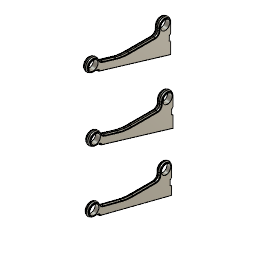
Shelf Brackets Filament Spool Holders A6 (Autodesk Fusion 360 design; units mm, degrees)
Autodesk Fusion 360 part; units mm, degrees
(part 1 of 2)
sketch "Sketch1" plane through (0, 0, 0) normal (1, 0, 0) x (0, 1, 0) in component "GROUND Spool Bambu Lab 1kg"
  circle A0 centre (0, 0) radius 27.5
  circle A1 centre (0, 0) radius 25
  circle A2 centre (0, 0) radius 100
  circle A3 centre (0, 0) radius 44.5
  circle A4 centre (0, 0) radius 41
  dimension "d1" = 55
  dimension "d2" = 50
  dimension "d3" = 200
  dimension "d4" = 89
  dimension "d5" = 82
  constraint coincident A0.centre A1.centre
  constraint concentric A1 A2
  constraint concentric A0 A3
  constraint concentric A0 A4
  measures "d1" diameter of A0
  measures "d2" diameter of A1
  measures "d3" diameter of A2
  measures "d4" diameter of A3
  measures "d5" diameter of A4
extrude "Extrude1" add sketch "Sketch1" against normal blind 3.5 contours A0 | A2 | A3 | A4 picked at (26.471206, -2.60824) picked at (80.962018, -7.178869) picked at (43.015012, -4.247705) picked at (36.347355, -2.036911) makes body 1 in component "GROUND Spool Bambu Lab 1kg"
extrude "Extrude2" add sketch "Sketch1" along normal blind 3.5 from surface at 60 separate body contours A0 | A2 | A3 | A4 picked at (26.471206, -2.60824) picked at (80.962018, -7.178869) picked at (43.015012, -4.247705) picked at (36.347355, -2.036911) makes body 2 in component "GROUND Spool Bambu Lab 1kg"
extrude "Extrude3" add sketch "Sketch1" along normal blind 63.5 contours A4 picked at (36.347355, -2.036911) bodies 1 2 in component "GROUND Spool Bambu Lab 1kg"
extrude "Extrude4" add sketch "Sketch1" along normal blind 32 contours A0 picked at (26.471206, -2.60824) bodies 1 in component "GROUND Spool Bambu Lab 1kg"
extrude "Extrude5" add sketch "Sketch1" along normal blind 60 separate body contours A3 picked at (43.015012, -4.247705) makes body 3 in component "GROUND Spool Bambu Lab 1kg"
sketch "Sketch1 (2)" plane through (0, 0, 0) normal (1, 0, 0) x (0, 1, 0) in component "Spool Bambu Lab 1kg (1)"
  circle A0 centre (0, 0) radius 27.5
  circle A1 centre (0, 0) radius 25
  circle A2 centre (0, 0) radius 100
  circle A3 centre (0, 0) radius 44.5
  circle A4 centre (0, 0) radius 41
  dimension "d1_1" = 55
  dimension "d2_1" = 50
  dimension "d3_1" = 200
  dimension "d4_1" = 89
  dimension "d5_1" = 82
  constraint coincident A0.centre A1.centre
  constraint concentric A1 A2
  constraint concentric A0 A3
  constraint concentric A0 A4
  measures "d1_1" diameter of A0
  measures "d2_1" diameter of A1
  measures "d3_1" diameter of A2
  measures "d4_1" diameter of A3
  measures "d5_1" diameter of A4
extrude "Extrude1'" add sketch "Sketch1 (2)" against normal blind 3.5 separate body contours A0 | A2 | A3 | A4 picked at (26.471206, -2.60824) picked at (80.962018, -7.178869) picked at (43.015012, -4.247705) picked at (36.347355, -2.036911) makes body 4 in component "Spool Bambu Lab 1kg (1)"
extrude "Extrude2'" add sketch "Sketch1 (2)" along normal blind 3.5 from surface at 60 separate body contours A0 | A2 | A3 | A4 picked at (26.471206, -2.60824) picked at (80.962018, -7.178869) picked at (43.015012, -4.247705) picked at (36.347355, -2.036911) makes body 5 in component "Spool Bambu Lab 1kg (1)"
extrude "Extrude3'" add sketch "Sketch1 (2)" along normal blind 63.5 contours A4 picked at (36.347355, -2.036911) bodies 4 5 in component "Spool Bambu Lab 1kg (1)"
extrude "Extrude4'" add sketch "Sketch1 (2)" along normal blind 32 contours A0 picked at (26.471206, -2.60824) bodies 4 in component "Spool Bambu Lab 1kg (1)"
extrude "Extrude5'" add sketch "Sketch1 (2)" along normal blind 60 separate body contours A3 picked at (43.015012, -4.247705) makes body 6 in component "Spool Bambu Lab 1kg (1)"
sketch "Sketch1 (3)" plane through (0, 0, 0) normal (1, 0, 0) x (0, 1, 0) in component "Box Bambu Lab Refill"
  line L0 (100, -97.5) -> (-100, -97.5)
  line L1 (-100, -97.5) -> (-100, 97.5)
  line L2 (-100, 97.5) -> (100, 97.5)
  line L3 (100, 97.5) -> (100, -97.5)
  line L4 (100, -97.5) -> (-100, 97.5) construction
  line L5 (-100, -97.5) -> (100, 97.5) construction
  dimension "d17" = 200
  dimension "d18" = 195
  constraint horizontal L0
  constraint perpendicular L0 L1
  constraint parallel L0 L2
  constraint parallel L1 L3
  constraint coincident L4 origin
  constraint coincident L5 origin
  measures "d17" distance of L1.end L2.end
  measures "d18" distance of L0.end L1.end
extrude "Extrude1''" add sketch "Sketch1 (3)" along normal blind 66 separate body contours L0 L1 L2 L3 picked at (33.333333, -32.5) makes body 7 in component "Box Bambu Lab Refill"
sketch "Sketch1 (4)" plane through (0, 0, 0) normal (1, 0, 0) x (0, 1, 0) in component "Box Bambu Lab with Spool"
  line L0 (110, -103) -> (-110, -103)
  line L1 (-110, -103) -> (-110, 103)
  line L2 (-110, 103) -> (110, 103)
  line L3 (110, 103) -> (110, -103)
  line L4 (110, -103) -> (-110, 103) construction
  line L5 (-110, -103) -> (110, 103) construction
  dimension "d17_1" = 220
  dimension "d18_1" = 206
  constraint horizontal L0
  constraint perpendicular L0 L1
  constraint parallel L0 L2
  constraint parallel L1 L3
  constraint coincident L4 origin
  constraint coincident L5 origin
  measures "d17_1" distance of L1.end L2.end
  measures "d18_1" distance of L0.end L1.end
extrude "Extrude1'''" add sketch "Sketch1 (4)" along normal blind 70 separate body contours L0 L1 L2 L3 picked at (36.666667, 34.333333) makes body 8 in component "Box Bambu Lab with Spool"
sketch "Sketch1 (5)" plane through (0, 0, 0) normal (1, 0, 0) x (0, 1, 0) in component "Box Polymaker"
  line L0 (111.5, -103.5) -> (-111.5, -103.5)
  line L1 (-111.5, -103.5) -> (-111.5, 103.5)
  line L2 (-111.5, 103.5) -> (111.5, 103.5)
  line L3 (111.5, 103.5) -> (111.5, -103.5)
  line L4 (111.5, -103.5) -> (-111.5, 103.5) construction
  line L5 (-111.5, -103.5) -> (111.5, 103.5) construction
  dimension "d25" = 223
  dimension "d26" = 207
  constraint horizontal L0
  constraint perpendicular L0 L1
  constraint parallel L0 L2
  constraint parallel L1 L3
  constraint coincident L4 origin
  constraint coincident L5 origin
  measures "d25" distance of L1.end L2.end
  measures "d26" distance of L0.end L1.end
extrude "Extrude1''''" add sketch "Sketch1 (5)" along normal blind 74 separate body contours L0 L1 L2 L3 picked at (37.166667, -34.5) makes body 9 in component "Box Polymaker"
sketch "Sketch1 (6)" plane through (0, 0, 0) normal (0, 1, 0) x (1, 0, 0) in component "Shelf Vertical Track 48\""
  line L0 (11.5, -624) -> (-11.5, -624)
  line L1 (-11.5, -624) -> (-11.5, 624)
  line L2 (-11.5, 624) -> (11.5, 624)
  line L3 (11.5, 624) -> (11.5, -624)
  line L4 (11.5, -624) -> (-11.5, 624) construction
  line L5 (-11.5, -624) -> (11.5, 624) construction
  line L6 (9.6, -624) -> (9.6, 624)
  line L7 (-9.6, 624) -> (-9.6, -624)
  line L8 (-3.75, -616.3) -> (-3.75, -600.3)
  arc A0 (-3.75, -600.3) -> (-6.75, -600.3) centre (-5.25, -600.3) ccw
  line L9 (-6.75, -600.3) -> (-6.75, -616.3)
  arc A1 (-6.75, -616.3) -> (-3.75, -616.3) centre (-5.25, -616.3) ccw
  line L10 (-5.25, -616.3) -> (-5.25, -600.3) construction
  line L11 (3.75, -600.3) -> (3.75, -616.3)
  line L12 (5.25, -616.3) -> (5.25, -600.3) construction
  arc A2 (3.75, -616.3) -> (6.75, -616.3) centre (5.25, -616.3) ccw
  line L13 (6.75, -616.3) -> (6.75, -600.3)
  arc A3 (6.75, -600.3) -> (3.75, -600.3) centre (5.25, -600.3) ccw
  line L14 (-5.25, -616.3) -> (5.25, -616.3) construction
  line L15 (0, -624) -> (0, 624) construction
  circle A4 centre (0, -591) radius 3
  circle A5 centre (0, -336.5) radius 3
  circle A6 centre (0, 107.5) radius 3
  circle A7 centre (0, 552) radius 3
  point P0 (0, -616.3)
  point P1 (0, -624)
  dimension "d29" = 23
  dimension "d30" = 1248
  dimension "d31" = 1.9
  dimension "d32" = 1.9
  dimension "d34" = 3
  dimension "d35" = 16
  dimension "d36" = 7.7
  dimension "d37" = 3
  dimension "d38" = 16
  dimension "d39" = 10.5
  dimension "d40" = 6
  dimension "d41" = 33
  dimension "d42" = 6
  dimension "d43" = 287.5
  dimension "d45" = 6
  dimension "d46" = 731.5
  dimension "d47" = 6
  dimension "d48" = 72
  constraint horizontal L0
  constraint perpendicular L0 L1
  constraint parallel L0 L2
  constraint parallel L1 L3
  constraint coincident L4 origin
  constraint coincident L5 origin
  constraint coincident L0 L6.start
  constraint coincident L2 L6.end
  constraint perpendicular L2 L6
  constraint coincident L2 L7.start
  constraint coincident L0 L7.end
  constraint perpendicular L0 L7
  constraint tangent L8 A0
  constraint tangent A0 L9
  constraint parallel L8 L9
  constraint tangent L9 A1
  constraint tangent L8 A1
  constraint vertical L10
  constraint tangent L13 A3
  constraint tangent L11 A3
  constraint parallel L11 L13
  constraint tangent L11 A2
  constraint tangent A2 L13
  constraint vertical L12
  constraint coincident A1.centre L10.start
  constraint coincident L12.start A2.centre
  constraint horizontal L14
  constraint midpoint L14 P0
  constraint midpoint L0 P1
  constraint coincident P1 L15.start
  constraint midpoint L2 L15.end
  constraint coincident P0 L15
  constraint coincident L15 A4.centre
  constraint coincident L15 A5.centre
  constraint coincident L15 A6.centre
  constraint coincident L15 A7.centre
  measures "d29" distance of L1.end L2.end
  measures "d30" distance of L0.end L1.end
  measures "d31" distance of L1 L7
  measures "d32" distance of L3 L6
  measures "d34" distance of L8 L9
  measures "d35" distance of A1.centre A0.centre
  measures "d36" distance of L0 A1.centre
  measures "d37" distance of L11 L13
  measures "d38" distance of L12.start L12.end
  measures "d39" distance of A1.centre L12.start
  measures "d40" diameter of A4
  measures "d41" distance of L0 A4.centre
  measures "d42" diameter of A5
  measures "d43" distance of L0 A5.centre
  measures "d45" diameter of A6
  measures "d46" distance of L0 A6.centre
  measures "d47" diameter of A7
  measures "d48" distance of L2 A7.centre
extrude "Extrude1'''''" add sketch "Sketch1 (6)" against normal blind 1.9 separate body contours L0 L2 L3 L6 | L0 L2 L6 L7 | L0 L1 L2 L7 picked at (10.866667, 208) picked at (0, 601) picked at (-10.233333, 208) makes body 10 in component "Shelf Vertical Track 48\""
extrude "Extrude2''" add sketch "Sketch1 (6)" along normal blind 15 contours L0 L2 L3 L6 | L0 L1 L2 L7 picked at (10.866667, 208) picked at (-10.233333, 208) bodies 10 in component "Shelf Vertical Track 48\""
fillet "Fillet1" radius 2 2 edges at (-11.5, -1.9, 0) (11.5, -1.9, 0) on bodies 10 in component "Shelf Vertical Track 48\""
fillet "Fillet2" radius 0.6 2 edges at (-9.6, 0, 0) (9.6, 0, 0) on bodies 10 in component "Shelf Vertical Track 48\""
pattern_linear "R-Pattern1" count 39 spacing 31.757896 along (0, 0, -1) of 8 faces at (6.75, -1.266667, 610.966667) (4.436181, -1.266667, 617.560039) (6.063819, -1.266667, 599.039961) (-4.436181, -1.266667, 599.039961) (-3.75, -1.266667, 610.966667) (-6.063819, -1.266667, 617.560039) (-6.75, -1.266667, 605.633333) (3.75, -1.266667, 605.633333) on bodies 10 in component "Shelf Vertical Track 48\""
sketch "Sketch1 (7)" plane through (0, 0, 0) normal (1, 0, 0) x (0, 1, 0) in component "Shelf Bracket 9.53\""
  line L0 (0, 0) -> (-265, 0)
  line L1 (0, 0) -> (0, -56) construction
  line L2 (0, -56) -> (-265, 0)
  line L3 (-242, 0) -> (-242, -4.860377)
  line L4 (-10, 0) -> (-10, -53.886792) construction
  line L5 (-12, 0) -> (-12, -53.464151) construction
  line L6 (-13, 0) -> (-13, -53.25283) construction
  line L7 (-11, 0) -> (-11, -53.675472) construction
  line L8 (0, -16.675472) -> (-10, -16.675472)
  line L9 (-4.5, -42.175472) -> (-11, -42.175472)
  line L10 (-8, -25.675472) -> (-12, -25.675472)
  line L11 (-8, -25.675472) -> (-4.5, -42.175472)
  line L12 (-12, -25.675472) -> (-12, -18.675472)
  line L13 (-13, -16.675472) -> (-13, -11.675472)
  line L14 (-13, -11.675472) -> (-10, -11.675472)
  line L15 (-10, -11.675472) -> (-10, -16.675472)
  line L16 (-12, -18.675472) -> (-13, -16.675472)
  line L17 (-11, -42.175472) -> (-11, -53.675472)
  line L18 (-255.810366, 0) -> (-11, -51.733511)
  line L19 (0, 0) -> (0, -16.675472)
  line L20 (-243.9, 0) -> (-243.9, -4.458868)
  point P0 (-242, 0)
  dimension "d65" = 265
  dimension "d66" = 56
  dimension "d67" = 242
  dimension "d68" = 10
  dimension "d69" = 12
  dimension "d70" = 13
  dimension "d71" = 11
  dimension "d72" = 37
  dimension "d73" = 11.5
  dimension "d74" = 28
  dimension "d75" = 6.5
  dimension "d76" = 4
  dimension "d77" = 7
  dimension "d78" = 9
  dimension "d79" = 14
  dimension "d82" = 1.9
  dimension "d88" = 1.9
  constraint coincident L0.start L1.start
  constraint horizontal L0
  constraint perpendicular L0 L1
  constraint coincident L0 P0
  constraint coincident P0 L3.start
  constraint perpendicular L0 L3
  constraint coincident L0 L4.start
  constraint perpendicular L0 L4
  constraint coincident L0 L5.start
  constraint perpendicular L0 L5
  constraint coincident L0 L6.start
  constraint perpendicular L0 L6
  constraint coincident L0 L7.start
  constraint perpendicular L0 L7
  constraint perpendicular L4 L8
  constraint perpendicular L7 L9
  constraint perpendicular L5 L10
  constraint perpendicular L10 L12
  constraint perpendicular L4 L14
  constraint parallel L2 L18
  constraint coincident L0 L20.start
  constraint perpendicular L0 L20
  measures "d65" distance of L0.start L0.end
  measures "d66" distance of L0.start L1.end
  measures "d67" distance of L1 P0
  measures "d68" distance of L1 L4
  measures "d69" distance of L1 L5
  measures "d70" distance of L1 L6
  measures "d71" distance of L1 L7
  measures "d82" distance of L2 L18
  measures "d88" distance of L3 L20
extrude "Extrude1''''''" add sketch "Sketch1 (7)" against normal blind 1.9 separate body contours L0 L3 L8 L9 L10 L11 L12 L13 L14 L15 L16 L17 L18 L19 | L0 L3 L18 L20 | L2 L3 L17 L18 | L2 L3 L18 L20 picked at (-88.333333, -23.589787) picked at (-242.633333, -1.811775) picked at (-165, -19.837435) picked at (-242.633333, -4.079221) makes body 11 in component "Shelf Bracket 9.53\""
extrude "Extrude2'''" add sketch "Sketch1 (7)" along normal blind 9.94 contours L0 L3 L18 L20 | L2 L3 L17 L18 | L2 L3 L18 L20 picked at (-242.633333, -1.811775) picked at (-165, -19.837435) picked at (-242.633333, -4.079221) bodies 11 in component "Shelf Bracket 9.53\""
extrude "Extrude3''" add sketch "Sketch1 (7)" along normal blind 1.9 from surface at 9.94 contours L0 L3 L8 L9 L10 L11 L12 L13 L14 L15 L16 L17 L18 L19 | L0 L3 L18 L20 | L2 L3 L17 L18 | L2 L3 L18 L20 picked at (-88.333333, -23.589787) picked at (-242.633333, -1.811775) picked at (-165, -19.837435) picked at (-242.633333, -4.079221) bodies 11 in component "Shelf Bracket 9.53\""
fillet "Fillet1'" radius 4 1 edges at (4.97, -242, -2.918417) on bodies 11 in component "Shelf Bracket 9.53\""
fillet "Fillet2'" radius 6 1 edges at (4.97, -243.9, -4.458868) on bodies 11 in component "Shelf Bracket 9.53\""
fillet "Fillet3" radius 1.8 4 edges at (10.89, 0, -16.675472) (-0.95, 0, -16.675472) (10.89, -10, -16.675472) (-0.95, -10, -16.675472) on bodies 11 in component "Shelf Bracket 9.53\""
fillet "Fillet4" radius 7 2 edges at (-0.95, 0, 0) (10.89, 0, 0) on bodies 11 in component "Shelf Bracket 9.53\""
fillet "Fillet5" radius 1.5 2 edges at (10.89, -8, -25.675472) (-0.95, -8, -25.675472) on bodies 11 in component "Shelf Bracket 9.53\""
fillet "Fillet6" radius 1.5 2 edges at (10.89, -4.5, -42.175472) (-0.95, -4.5, -42.175472) on bodies 11 in component "Shelf Bracket 9.53\""
fillet "Fillet7" radius 0.6 12 edges at (10.89, -10, -11.675472) (10.89, -13, -11.675472) (-0.95, -13, -11.675472) (-0.95, -10, -11.675472) (-0.95, -13, -16.675472) (10.89, -13, -16.675472) (10.89, -12, -18.675472) (-0.95, -12, -18.675472) (10.89, -12, -25.675472) (-0.95, -12, -25.675472) (10.89, -11, -42.175472) (-0.95, -11, -42.175472) on bodies 11 in component "Shelf Bracket 9.53\""
fillet "Fillet8" radius 0.8 1 edges at (4.97, -11, -53.675472) on bodies 11 in component "Shelf Bracket 9.53\""
sketch "Sketch2" plane through (0, -11.32809, -53.60614) normal (0, -0.206755, -0.978393) x (1, 0, 0) in component "Shelf Bracket 9.53\""
  line L0 (-1.9, 0.651389) -> (11.84, 0.651389)
  line L1 (11.84, 0.651389) -> (11.84, 232.857773)
  line L2 (11.84, 232.857773) -> (-1.9, 232.857773)
  line L3 (-1.9, 232.857773) -> (-1.9, 0.651389)
  line L4 (4.97, 232.857773) -> (4.97, 0.651389) construction
  circle A0 centre (4.97, 62.651389) radius 2
  line L5 (2.97, 163.651389) -> (2.97, 148.651389)
  arc A1 (2.97, 148.651389) -> (6.97, 148.651389) centre (4.97, 148.651389) ccw
  line L6 (6.97, 148.651389) -> (6.97, 163.651389)
  arc A2 (6.97, 163.651389) -> (2.97, 163.651389) centre (4.97, 163.651389) ccw
  line L7 (4.97, 163.651389) -> (4.97, 148.651389) construction
  dimension "d105" = 4
  dimension "d106" = 62
  dimension "d107" = 4
  dimension "d108" = 15
  dimension "d109" = 148
  constraint tangent L5 A1
  constraint tangent A1 L6
  constraint parallel L5 L6
  constraint tangent L6 A2
  constraint tangent L5 A2
  constraint parallel L4 L7
  measures "d105" diameter of A0
  measures "d107" distance of L5 L6
extrude "Extrude4''" cut sketch "Sketch2" against normal up to surface (1.9 mm away) contours A0 | L5 A1 L6 A2 picked at (5.466147, 63.005476) picked at (4.303333, 158.651389) bodies 11 in component "Shelf Bracket 9.53\""
sketch "Sketch1 (8)" plane through (0, 0, 0) normal (1, 0, 0) x (0, 1, 0) in component "Lowes Shelf Bracket 9.53\" (1)"
  line L0 (0, 0) -> (-188.527967, 0)
  line L1 (-11, -53.2) -> (-188.527967, 0)
  line L2 (-174, 0) -> (-174, -4.353612)
  line L3 (-10, 0) -> (-10, -12) construction
  line L4 (-12, 0) -> (-12, -52.900329) construction
  line L5 (-13, 0) -> (-13, -52.600658) construction
  line L6 (-11, 0) -> (-11, -53.2) construction
  line L7 (0, -16.6) -> (-10, -16.6)
  line L8 (-4.5, -42.1) -> (-11, -42.1)
  line L9 (-8, -26) -> (-12, -26)
  line L10 (-8, -26) -> (-4.5, -42.1)
  line L11 (-12, -26) -> (-12, -19)
  line L12 (-13, -17) -> (-13, -12)
  line L13 (-13, -12) -> (-10, -12)
  line L14 (-10, -12) -> (-10, -16.6)
  line L15 (-12, -19) -> (-13, -17)
  line L16 (-11, -42.1) -> (-11, -53.2)
  line L17 (-184.417312, 0) -> (-11, -51.968155)
  line L18 (0, 0) -> (0, -16.6)
  line L19 (-175.18, 0) -> (-175.18, -4)
  point P0 (-174, 0)
  point P1 (-175.18, -4)
  dimension "d75_1" = 6.5
  dimension "d76_1" = 4
  dimension "d77_1" = 7
  dimension "d78_1" = 9
  dimension "d79_1" = 14
  dimension "d82_1" = 1.18
  dimension "d88_1" = 1.18
  dimension "d198" = 4
  dimension "d199" = 53.2
  dimension "d200" = 16.6
  dimension "d201" = 12
  dimension "d202" = 42.1
  dimension "d203" = 10
  dimension "d204" = 11
  dimension "d205" = 12
  dimension "d206" = 13
  dimension "d207" = 174
  constraint coincident L0.start L18.start
  constraint horizontal L0
  constraint coincident L0 P0
  constraint coincident P0 L2.start
  constraint perpendicular L0 L2
  constraint coincident L0 L3.start
  constraint perpendicular L0 L3
  constraint coincident L0 L4.start
  constraint perpendicular L0 L4
  constraint coincident L0 L5.start
  constraint perpendicular L0 L5
  constraint coincident L0 L6.start
  constraint perpendicular L0 L6
  constraint coincident L1 L6.end
  constraint coincident L3 L7.end
  constraint perpendicular L3 L7
  constraint coincident L6 L8.end
  constraint perpendicular L6 L8
  constraint coincident L4 L9.end
  constraint perpendicular L4 L9
  constraint perpendicular L9 L11
  constraint coincident L5 L12.start
  constraint coincident L5 L12.end
  constraint coincident L3 L13.end
  constraint perpendicular L3 L13
  constraint parallel L1 L17
  constraint coincident L0 L19.start
  constraint perpendicular L0 L19
  constraint coincident L1 P1
  constraint coincident L19 P1
  constraint coincident L1.start L6
  constraint coincident L3.end L13.end
  measures "d75_1" distance of L8.start L8.end
  measures "d76_1" distance of L9.start L9.end
  measures "d77_1" distance of L9.end L11.end
  measures "d78_1" vertical distance of L9.end L12.start
  measures "d79_1" vertical distance of L9.end L12.end
  measures "d82_1" distance of L1 L17
  measures "d88_1" distance of L2 L19
  measures "d198" distance of L19.start P1
  measures "d199" distance of L0 L1.start
  measures "d200" distance of L0 L7
  measures "d201" distance of L0 L13
  measures "d202" distance of L0 L8
  measures "d203" distance of L3 L18
  measures "d204" distance of L6 L18
  measures "d205" distance of L4 L18
  measures "d206" distance of L5 L18
  measures "d207" distance of L2 L18
extrude "Extrude1'''''''" add sketch "Sketch1 (8)" against normal blind 1.18 separate body contours L0 L2 L7 L8 L9 L10 L11 L12 L13 L14 L15 L16 L17 L18 | L0 L2 L17 L19 | L1 L2 L16 L17 | L1 L2 L17 L19 picked at (-65.666667, -23.740589) picked at (-174.393333, -1.963307) picked at (-65.333333, -36.507256) picked at (-174.393333, -3.825126) makes body 12 in component "Lowes Shelf Bracket 9.53\" (1)"
extrude "Extrude2''''" add sketch "Sketch1 (8)" along normal blind 10.64 contours L0 L2 L17 L19 | L1 L2 L16 L17 | L1 L2 L17 L19 picked at (-174.393333, -1.963307) picked at (-65.333333, -36.507256) picked at (-174.393333, -3.825126) bodies 12 in component "Lowes Shelf Bracket 9.53\" (1)"
extrude "Extrude3'''" add sketch "Sketch1 (8)" along normal blind 1.18 from surface at 10.64 contours L0 L2 L7 L8 L9 L10 L11 L12 L13 L14 L15 L16 L17 L18 | L0 L2 L17 L19 | L1 L2 L16 L17 | L1 L2 L17 L19 picked at (-65.666667, -23.740589) picked at (-174.393333, -1.963307) picked at (-65.333333, -36.507256) picked at (-174.393333, -3.825126) bodies 12 in component "Lowes Shelf Bracket 9.53\" (1)"
fillet "Fillet1''" radius 4 1 edges at (5.32, -174, -3.121767) on bodies 12 in component "Lowes Shelf Bracket 9.53\" (1)"
fillet "Fillet2''" radius 6 1 edges at (5.32, -175.18, -4) on bodies 12 in component "Lowes Shelf Bracket 9.53\" (1)"
fillet "Fillet3'" radius 1.8 4 edges at (11.23, 0, -16.6) (-0.59, 0, -16.6) (11.23, -10, -16.6) (-0.59, -10, -16.6) on bodies 12 in component "Lowes Shelf Bracket 9.53\" (1)"
fillet "Fillet4'" radius 7 2 edges at (-0.59, 0, 0) (11.23, 0, 0) on bodies 12 in component "Lowes Shelf Bracket 9.53\" (1)"
fillet "Fillet5'" radius 1.5 2 edges at (11.23, -8, -26) (-0.59, -8, -26) on bodies 12 in component "Lowes Shelf Bracket 9.53\" (1)"
fillet "Fillet6'" radius 1.5 2 edges at (11.23, -4.5, -42.1) (-0.59, -4.5, -42.1) on bodies 12 in component "Lowes Shelf Bracket 9.53\" (1)"
fillet "Fillet7'" radius 0.6 12 edges at (11.23, -10, -12) (11.23, -13, -12) (-0.59, -13, -12) (-0.59, -10, -12) (-0.59, -13, -17) (11.23, -13, -17) (11.23, -12, -19) (-0.59, -12, -19) (11.23, -12, -26) (-0.59, -12, -26) (11.23, -11, -42.1) (-0.59, -11, -42.1) on bodies 12 in component "Lowes Shelf Bracket 9.53\" (1)"
fillet "Fillet8'" radius 0.8 1 edges at (5.32, -11, -53.2) on bodies 12 in component "Lowes Shelf Bracket 9.53\" (1)"
sketch "Sketch2 (2)" plane through (0, -15.535226, -51.840924) normal (0, -0.287059, -0.957913) x (1, 0, 0) in component "Lowes Shelf Bracket 9.53\" (1)"
  line L0 (-1.18, -3.659601) -> (11.82, -3.659601)
  line L1 (11.82, -3.659601) -> (11.82, 162.212706)
  line L2 (11.82, 162.212706) -> (-1.18, 162.212706)
  line L3 (-1.18, 162.212706) -> (-1.18, -3.659601)
  line L4 (5.32, 162.212706) -> (5.32, -3.659601) construction
  circle A0 centre (5.32, 41.840399) radius 2
  line L5 (3.32, 116.840399) -> (3.32, 101.840399)
  arc A1 (3.32, 101.840399) -> (7.32, 101.840399) centre (5.32, 101.840399) ccw
  line L6 (7.32, 101.840399) -> (7.32, 116.840399)
  arc A2 (7.32, 116.840399) -> (3.32, 116.840399) centre (5.32, 116.840399) ccw
  line L7 (5.32, 116.840399) -> (5.32, 101.840399) construction
  dimension "d105_1" = 4
  dimension "d106_1" = 45.5
  dimension "d107_1" = 4
  dimension "d108_1" = 15
  dimension "d109_1" = 105.5
  constraint tangent L5 A1
  constraint tangent A1 L6
  constraint parallel L5 L6
  constraint tangent L6 A2
  constraint tangent L5 A2
  constraint parallel L4 L7
  measures "d105_1" diameter of A0
  measures "d107_1" distance of L5 L6
extrude "Extrude4'''" cut sketch "Sketch2 (2)" against normal up to surface (1.18 mm away) contours A0 | L5 A1 L6 A2 picked at (5.847074, 41.218829) picked at (5.986667, 106.840399) bodies 12 in component "Lowes Shelf Bracket 9.53\" (1)"
sketch "Sketch1 (9)" plane through (0, 0, 0) normal (1, 0, 0) x (0, 1, 0) in component "Pipe Holder"
  arc A0 (-12, -18.817112) -> (-12.063344, -18.548784) centre (-12.6, -18.817112) ccw
  line L0 (-12.063344, -18.548784) -> (-12.936656, -16.802159)
  arc A1 (-13, -16.533831) -> (-12.936656, -16.802159) centre (-12.4, -16.533831) ccw
  line L1 (-13, -16.533831) -> (-13, -12.275472)
  arc A2 (-12.4, -11.675472) -> (-13, -12.275472) centre (-12.4, -12.275472) ccw
  line L2 (-12.4, -11.675472) -> (-10.6, -11.675472)
  arc A3 (-10, -12.275472) -> (-10.6, -11.675472) centre (-10.6, -12.275472) ccw
  line L3 (-10, -12.275472) -> (-10, -14.875472)
  arc A4 (-10, -14.875472) -> (-8.2, -16.675472) centre (-8.2, -14.875472) ccw
  line L4 (-8.2, -16.675472) -> (-1.8, -16.675472)
  arc A5 (-1.8, -16.675472) -> (0, -14.875472) centre (-1.8, -14.875472) ccw
  line L5 (0, -14.875472) -> (0, -7)
  arc A6 (0, -7) -> (-7, 0) centre (-7, -7) ccw
  line L6 (-7, 0) -> (-242, 0)
  arc A7 (-242, 0) -> (-238.840446, -3.586096) centre (-238.013428, 0.327475) ccw
  line L7 (-238.840446, -3.586096) -> (-11, -51.733511)
  line L8 (-11, -51.733511) -> (-11, -42.775472)
  arc A8 (-10.4, -42.175472) -> (-11, -42.775472) centre (-10.4, -42.775472) ccw
  line L9 (-10.4, -42.175472) -> (-6.351557, -42.175472)
  arc A9 (-6.351557, -42.175472) -> (-4.884206, -40.364215) centre (-6.351557, -40.675472) ccw
  line L10 (-4.884206, -40.364215) -> (-7.747842, -26.864215)
  arc A10 (-7.747842, -26.864215) -> (-9.215193, -25.675472) centre (-9.215193, -27.175472) ccw
  line L11 (-9.215193, -25.675472) -> (-11.4, -25.675472)
  arc A11 (-12, -25.075472) -> (-11.4, -25.675472) centre (-11.4, -25.075472) ccw
  line L12 (-12, -25.075472) -> (-12, -18.817112)
  line L13 (-14, 0) -> (-14, -51.099549)
  line L14 (-237.013428, 0) -> (-237.013428, -3.972183)
  circle A12 centre (-27.8, 10.8) radius 9.8
  circle A13 centre (-27.8, 10.8) radius 13.8
  circle A14 centre (-228.013428, 12.8) radius 9.8
  circle A15 centre (-228.013428, 12.8) radius 13.8
  line L15 (-14, 0) -> (-14, 10.8)
  line L16 (-27.8, 10.8) -> (-27.8, -3) construction
  line L17 (-41.6, 0) -> (-41.6, 10.8)
  line L18 (-228.013428, 12.8) -> (-228.013428, -1) construction
  line L19 (-218.255354, 22.558074) -> (-195.69728, 0)
  line L20 (-237.013428, 0) -> (-237.013428, 1)
  line L21 (-237.013428, 1) -> (-243.74918, 1)
  arc A16 (-11.965404, -53.471462) -> (-11, -52.688748) centre (-11.8, -52.688748) ccw
  line L22 (-11.965404, -53.471462) -> (-239.154461, -5.461699)
  arc A17 (-243.9, 0) -> (-239.154461, -5.461699) centre (-237.913933, 0.408658) ccw
  line L23 (-243.9, 0) -> (-7, 0)
  arc A18 (0, -7) -> (-7, 0) centre (-7, -7) ccw
  line L24 (0, -7) -> (0, -14.875472)
  arc A19 (-1.8, -16.675472) -> (0, -14.875472) centre (-1.8, -14.875472) ccw
  line L25 (-1.8, -16.675472) -> (-8.2, -16.675472)
  arc A20 (-10, -14.875472) -> (-8.2, -16.675472) centre (-8.2, -14.875472) ccw
  line L26 (-10, -14.875472) -> (-10, -12.275472)
  arc A21 (-10, -12.275472) -> (-10.6, -11.675472) centre (-10.6, -12.275472) ccw
  line L27 (-10.6, -11.675472) -> (-12.4, -11.675472)
  arc A22 (-12.4, -11.675472) -> (-13, -12.275472) centre (-12.4, -12.275472) ccw
  line L28 (-13, -12.275472) -> (-13, -16.533831)
  arc A23 (-13, -16.533831) -> (-12.936656, -16.802159) centre (-12.4, -16.533831) ccw
  line L29 (-12.936656, -16.802159) -> (-12.063344, -18.548784)
  arc A24 (-12, -18.817112) -> (-12.063344, -18.548784) centre (-12.6, -18.817112) ccw
  line L30 (-12, -18.817112) -> (-12, -25.075472)
  arc A25 (-12, -25.075472) -> (-11.4, -25.675472) centre (-11.4, -25.075472) ccw
  line L31 (-11.4, -25.675472) -> (-9.215193, -25.675472)
  arc A26 (-7.747842, -26.864215) -> (-9.215193, -25.675472) centre (-9.215193, -27.175472) ccw
  line L32 (-7.747842, -26.864215) -> (-4.884206, -40.364215)
  arc A27 (-6.351557, -42.175472) -> (-4.884206, -40.364215) centre (-6.351557, -40.675472) ccw
  line L33 (-6.351557, -42.175472) -> (-10.4, -42.175472)
  arc A28 (-10.4, -42.175472) -> (-11, -42.775472) centre (-10.4, -42.775472) ccw
  line L34 (-11, -42.775472) -> (-11, -52.688748)
  line L35 (-243.9, 0) -> (-241.659102, 14.858047)
  line L36 (-237.013428, -3.972183) -> (-240.74918, 1)
  dimension "d114" = 1
  dimension "d115" = 1
  dimension "d116" = 19.6
  dimension "d117" = 27.6
  dimension "d118" = 19.6
  dimension "d119" = 27.6
  dimension "d123" = 1
  dimension "d124" = 45
  dimension "d153" = 10
  dimension "d160" = 3
  dimension "d161" = 1
  dimension "d163" = 3
  constraint coincident L6 L13.start
  constraint perpendicular L6 L13
  constraint perpendicular L6 L14
  constraint concentric A12 A13
  constraint concentric A14 A15
  constraint coincident A13 L15.end
  constraint coincident A12.centre A13.centre
  constraint coincident A13 L16.end
  constraint vertical L16
  constraint tangent A13 L15
  constraint vertical L15
  constraint coincident L6 L17.start
  constraint coincident A13 L17.end
  constraint vertical L17
  constraint tangent A13 L17
  constraint vertical L18
  constraint vertical L20
  constraint perpendicular L20 L21
  constraint tangent A15 L19
  constraint coincident A17.start L23.start
  constraint tangent A15 L35
  measures "d115" distance of L1 L13
  measures "d116" diameter of A12
  measures "d117" diameter of A13
  measures "d118" diameter of A14
  measures "d119" diameter of A15
  measures "d124" angle of L6 L19
  measures "d160" distance of L16.end L23
extrude "Extrude1''''''''" add sketch "Sketch1 (9)" along normal up to surface (9.94 mm away) separate body contours L6 L7 L13 L14 A13 A15 L23 | L6 L14 L23 L36 | L6 A13 L15 L23 | L6 A15 L20 L21 L23 L35 | L6 L20 L21 L23 L36 | L6 A13 L23 | L6 A13 L23 | L6 A15 L23 | L6 A15 L23 | L6 A13 L17 L23 | L6 A15 L19 L23 picked at (-83.76576, -17.033183) picked at (-238.008235, -1.324061) picked at (-16.032674, 1.473269) picked at (-241.317687, 2.361321) picked at (-239.253485, 0.666667) picked at (-25.503866, -0.385947) picked at (-36.069082, 1.513719) picked at (-228.257546, 1.009134) picked at (-229.175331, -0.184174) picked at (-39.567326, 1.473269) picked at (-208.691501, 5.205571) makes body 13 in component "Pipe Holder"
move_face "OffsetFaces1" offset -0.3 1 faces at (9.94, -83.76576, -17.033183) on bodies 13 in component "Pipe Holder"
move_face "OffsetFaces2" offset -0.3 1 faces at (0, -83.76576, -17.033183) on bodies 13 in component "Pipe Holder"
fillet "Fillet3''" radius 40 1 edges at (4.82, -195.69728, 0) on bodies 13 in component "Pipe Holder"
fillet "Fillet4''" radius 8 1 edges at (4.82, -41.6, 0) on bodies 13 in component "Pipe Holder"
fillet "Fillet6''" radius 1 3 edges at (4.97, -240.74918, 1) (4.97, -243.74918, 1) (4.97, -237.013428, -3.972183) on bodies 13 in component "Pipe Holder"
chamfer "Chamfer1" distance 1 angle 45 30 edges at (0.3, -125.323085, -27.574671) (0.3, -236.976815, -3.914727) (0.3, -238.844031, -1.5357) (0.3, -240.801815, 0.894617) (0.3, -241.917849, 1) (0.3, -243.345052, 1.347748) (0.3, -242.617484, 8.50359) (0.3, -232.326311, 25.908739) (0.3, -212.834182, 17.136901) (0.3, -194.436075, 3.044819) (0.3, -114.364369, 0) (0.3, -43.943146, 2.343146) (0.3, -41.6, 9.4) (0.3, -27.8, 24.6) (0.3, -14, -20.149775) (9.64, -125.323085, -27.574671) (9.64, -236.976815, -3.914727) (9.64, -238.844031, -1.5357) (9.64, -240.801815, 0.894617) (9.64, -241.917849, 1) (9.64, -243.345052, 1.347748) (9.64, -242.617484, 8.50359) (9.64, -232.326311, 25.908739) (9.64, -212.834182, 17.136901) (9.64, -194.436075, 3.044819) (9.64, -114.364369, 0) (9.64, -43.943146, 2.343146) (9.64, -41.6, 9.4) (9.64, -27.8, 24.6) (9.64, -14, -20.149775) on bodies 13 in component "Pipe Holder"
sketch "Sketch2 (3)" plane through (0, -10.935256, -51.747193) normal (0, -0.206755, -0.978393) x (1, 0, 0) in component "Pipe Holder"
  line L0 (6.97, 163.651389) -> (6.97, 148.651389)
  arc A0 (2.97, 148.651389) -> (6.97, 148.651389) centre (4.97, 148.651389) ccw
  line L1 (2.97, 148.651389) -> (2.97, 163.651389)
  arc A1 (6.97, 163.651389) -> (2.97, 163.651389) centre (4.97, 163.651389) ccw
  circle A2 centre (4.97, 62.651389) radius 2
  line L2 (-1.9, 0.651389) -> (11.84, 0.651389)
  line L3 (11.84, 0.651389) -> (11.84, 232.857773)
  line L4 (11.84, 232.857773) -> (-1.9, 232.857773)
  line L5 (-1.9, 232.857773) -> (-1.9, 0.651389)
  circle A3 centre (4.97, 62.651389) radius 1.7
  line L6 (4.97, 163.651389) -> (4.97, 148.651389) construction
  circle A4 centre (4.97, 156.151389) radius 1.7
  point P0 (4.97, 156.151389)
  dimension "d142" = 3.4
  dimension "d143" = 3.4
  constraint concentric A2 A3
  measures "d142" diameter of A3
  measures "d143" diameter of A4
extrude "Extrude2'''''" cut sketch "Sketch2 (3)" against normal blind 10 contours A3 | A4 picked at (5.461703, 62.488092) picked at (3.721887, 155.984361) bodies 13 in component "Pipe Holder"
sketch "Sketch1 (10)" plane through (0, 0, 0) normal (1, 0, 0) x (0, 1, 0) in component "Lowes Pipe Holder 6.75\""
  line L0 (-183.8, 14.828973) -> (-183.8, 1.028973) construction
  line L1 (-27.8, 12.828973) -> (-27.8, -0.971027) construction
  circle A0 centre (-183.8, 14.828973) radius 10.05
  circle A1 centre (-27.8, 12.828973) radius 10.05
  line L2 (-41.6, 0.028973) -> (-41.6, 12.828973)
  circle A2 centre (-183.8, 14.828973) radius 13.8
  line L3 (-14, 0.028973) -> (-14, -51.040169)
  line L4 (-14, 0.028973) -> (-14, 12.828973)
  circle A3 centre (-27.8, 12.828973) radius 13.8
  line L5 (-170, 14.828973) -> (-120.61252, 0.028973)
  arc A4 (-12.029647, -52.862472) -> (-11, -52.096141) centre (-11.8, -52.096141) ccw
  line L6 (-12.029647, -52.862472) -> (-170.920879, -5.247363)
  arc A5 (-175.18, 0.028973) -> (-170.920879, -5.247363) centre (-169.198527, 0.500115) ccw
  line L7 (-175.18, 0.028973) -> (-7, 0.028973)
  arc A6 (0, -6.971027) -> (-7, 0.028973) centre (-7, -6.971027) ccw
  line L8 (0, -6.971027) -> (0, -14.771027)
  arc A7 (-1.8, -16.571027) -> (0, -14.771027) centre (-1.8, -14.771027) ccw
  line L9 (-1.8, -16.571027) -> (-8.2, -16.571027)
  arc A8 (-10, -14.771027) -> (-8.2, -16.571027) centre (-8.2, -14.771027) ccw
  line L10 (-10, -14.771027) -> (-10, -12.571027)
  arc A9 (-10, -12.571027) -> (-10.6, -11.971027) centre (-10.6, -12.571027) ccw
  line L11 (-10.6, -11.971027) -> (-12.4, -11.971027)
  arc A10 (-12.4, -11.971027) -> (-13, -12.571027) centre (-12.4, -12.571027) ccw
  line L12 (-13, -12.571027) -> (-13, -16.829386)
  arc A11 (-13, -16.829386) -> (-12.936656, -17.097715) centre (-12.4, -16.829386) ccw
  line L13 (-12.936656, -17.097715) -> (-12.063344, -18.84434)
  arc A12 (-12, -19.112668) -> (-12.063344, -18.84434) centre (-12.6, -19.112668) ccw
  line L14 (-12, -19.112668) -> (-12, -25.371027)
  arc A13 (-12, -25.371027) -> (-11.4, -25.971027) centre (-11.4, -25.371027) ccw
  line L15 (-11.4, -25.971027) -> (-9.208948, -25.971027)
  arc A14 (-7.743184, -27.152383) -> (-9.208948, -25.971027) centre (-9.208948, -27.471027) ccw
  line L16 (-7.743184, -27.152383) -> (-4.895357, -40.252383)
  arc A15 (-6.361122, -42.071027) -> (-4.895357, -40.252383) centre (-6.361122, -40.571027) ccw
  line L17 (-6.361122, -42.071027) -> (-10.4, -42.071027)
  arc A16 (-10.4, -42.071027) -> (-11, -42.671027) centre (-10.4, -42.671027) ccw
  line L18 (-11, -42.671027) -> (-11, -52.096141)
  arc A17 (-12, -19.112668) -> (-12.063344, -18.84434) centre (-12.6, -19.112668) ccw
  line L19 (-12.063344, -18.84434) -> (-12.936656, -17.097715)
  arc A18 (-13, -16.829386) -> (-12.936656, -17.097715) centre (-12.4, -16.829386) ccw
  line L20 (-13, -16.829386) -> (-13, -12.571027)
  arc A19 (-12.4, -11.971027) -> (-13, -12.571027) centre (-12.4, -12.571027) ccw
  line L21 (-12.4, -11.971027) -> (-10.6, -11.971027)
  arc A20 (-10, -12.571027) -> (-10.6, -11.971027) centre (-10.6, -12.571027) ccw
  line L22 (-10, -12.571027) -> (-10, -14.771027)
  arc A21 (-10, -14.771027) -> (-8.2, -16.571027) centre (-8.2, -14.771027) ccw
  line L23 (-8.2, -16.571027) -> (-1.8, -16.571027)
  arc A22 (-1.8, -16.571027) -> (0, -14.771027) centre (-1.8, -14.771027) ccw
  line L24 (0, -14.771027) -> (0, -6.971027)
  arc A23 (0, -6.971027) -> (-7, 0.028973) centre (-7, -6.971027) ccw
  line L25 (-7, 0.028973) -> (-174, 0.028973)
  arc A24 (-174, -0.115734) -> (-171.148235, -3.947386) centre (-170, -0.115734) ccw
  line L26 (-171.148235, -3.947386) -> (-11, -51.939183)
  line L27 (-11, -51.939183) -> (-11, -42.671027)
  arc A25 (-10.4, -42.071027) -> (-11, -42.671027) centre (-10.4, -42.671027) ccw
  line L28 (-10.4, -42.071027) -> (-6.361122, -42.071027)
  arc A26 (-6.361122, -42.071027) -> (-4.895357, -40.252383) centre (-6.361122, -40.571027) ccw
  line L29 (-4.895357, -40.252383) -> (-7.743184, -27.152383)
  arc A27 (-7.743184, -27.152383) -> (-9.208948, -25.971027) centre (-9.208948, -27.471027) ccw
  line L30 (-9.208948, -25.971027) -> (-11.4, -25.971027)
  arc A28 (-12, -25.371027) -> (-11.4, -25.971027) centre (-11.4, -25.371027) ccw
  line L31 (-12, -25.371027) -> (-12, -19.112668)
  line L32 (-183.8, 14.828973) -> (-170, 14.828973) construction
  line L33 (-171.148235, -3.947386) -> (-174.021337, 1.028973)
  line L34 (-174.021337, 1.028973) -> (-183.8, 1.028973)
  line L35 (-174, 0.028973) -> (-174, -0.115734)
  line L36 (-14, -6.975529) -> (-19, -11.171027)
  line L37 (-19, -11.171027) -> (-19, -21.171027)
  line L38 (-19, -21.171027) -> (-14, -25.366525)
  point P0 (-19, -16.171027)
  dimension "d168" = 20.1
  dimension "d169" = 27.6
  dimension "d170" = 20.1
  dimension "d171" = 27.6
  dimension "d178" = 1
  dimension "d179" = 1
  dimension "d180" = 1
  dimension "d181" = 60
  dimension "d193" = 156
  dimension "d244" = 5
  dimension "d245" = 130
  dimension "d246" = 10
  dimension "d247" = 29
  constraint concentric A1 A3
  constraint concentric A0 A2
  constraint vertical L1
  constraint tangent L4 A3
  constraint vertical L4
  constraint vertical L2
  constraint tangent L2 A3
  constraint vertical L0
  constraint horizontal L32
  constraint parallel L7 L34
  constraint tangent A2 L34
  constraint parallel L5 L26
  constraint perpendicular L7 L37
  constraint equal L36 L38
  measures "d168" diameter of A1
  measures "d169" diameter of A3
  measures "d170" diameter of A0
  measures "d171" diameter of A2
  measures "d178" distance of L3 L12
  measures "d181" angle of L7 L33
  measures "d193" distance of L0 L1
  measures "d244" distance of L3 L37
  measures "d245" angle of L36 L37
extrude "Extrude1'''''''''" add sketch "Sketch1 (10)" along normal up to surface (10.64 mm away) separate body contours L3 A3 L7 L25 L26 L33 L36 L37 L38 | L2 A3 L7 L25 | A3 L7 L25 | A2 L5 L7 L25 L33 L34 | A3 L7 L25 | L4 A3 L7 L25 | A2 picked at (-58.737507, -16.994075) picked at (-38.681994, 1.87568) picked at (-28.050346, 0.955007) picked at (-155.101195, 3.051397) picked at (-26.638096, -0.155201) picked at (-16.918006, 1.87568) picked at (-184.725306, 2.338128) makes body 14 in component "Lowes Pipe Holder 6.75\""
move_face "OffsetFaces1'" offset -0.3 1 faces at (0, -58.737507, -16.994075) on bodies 14 in component "Lowes Pipe Holder 6.75\""
move_face "OffsetFaces2'" offset -0.3 1 faces at (10.64, -58.737507, -16.994075) on bodies 14 in component "Lowes Pipe Holder 6.75\""
fillet "Fillet1'''" radius 8 1 edges at (5.32, -41.6, 0.028973) on bodies 14 in component "Lowes Pipe Holder 6.75\""
fillet "Fillet2'''" radius 100 1 edges at (5.32, -120.61252, 0.028973) on bodies 14 in component "Lowes Pipe Holder 6.75\""
fillet "Fillet3'''" radius 10 1 edges at (5.32, -170, 14.828973) on bodies 14 in component "Lowes Pipe Holder 6.75\""
fillet "Fillet4'''" radius 3 2 edges at (5.32, -174.021337, 1.028973) (5.32, -171.148235, -3.947386) on bodies 14 in component "Lowes Pipe Holder 6.75\""
chamfer "Chamfer1'" distance 2 angle 45 30 edges at (0.3, -92.003508, -27.664773) (0.3, -171.00686, -3.768636) (0.3, -172.449614, -1.693332) (0.3, -174.253388, 0.627049) (0.3, -179.776694, 1.028973) (0.3, -195.051214, 22.819603) (0.3, -168.240424, 15.442932) (0.3, -149.428084, 8.664164) (0.3, -120.457436, 1.086743) (0.3, -77.775525, 0.028973) (0.3, -43.943146, 2.372118) (0.3, -41.6, 10.428973) (0.3, -27.8, 26.628973) (0.3, -14, -38.203347) (0.3, -14, 2.926722) (10.34, -92.003508, -27.664773) (10.34, -171.00686, -3.768636) (10.34, -172.449614, -1.693332) (10.34, -174.253388, 0.627049) (10.34, -179.776694, 1.028973) (10.34, -195.051214, 22.819603) (10.34, -168.240424, 15.442932) (10.34, -149.428084, 8.664164) (10.34, -120.457436, 1.086743) (10.34, -77.775525, 0.028973) (10.34, -43.943146, 2.372118) (10.34, -41.6, 10.428973) (10.34, -27.8, 26.628973) (10.34, -14, -38.203347) (10.34, -14, 2.926722) on bodies 14 in component "Lowes Pipe Holder 6.75\""
fillet "Fillet5''" radius 4 30 edges at (2.3, -92.003508, -27.664773) (2.3, -171.00686, -3.768636) (2.3, -172.449614, -1.693332) (2.3, -174.253388, 0.627049) (2.3, -179.776694, 1.028973) (2.3, -195.051214, 22.819603) (2.3, -168.240424, 15.442932) (2.3, -149.428084, 8.664164) (2.3, -120.457436, 1.086743) (2.3, -77.775525, 0.028973) (2.3, -43.943146, 2.372118) (2.3, -41.6, 10.428973) (2.3, -27.8, 26.628973) (2.3, -14, 2.926722) (2.3, -14, -38.203347) (8.34, -14, 2.926722) (8.34, -14, -38.203347) (8.34, -27.8, 26.628973) (8.34, -41.6, 10.428973) (8.34, -43.943146, 2.372118) (8.34, -77.775525, 0.028973) (8.34, -120.457436, 1.086743) (8.34, -149.428084, 8.664164) (8.34, -168.240424, 15.442932) (8.34, -195.051214, 22.819603) (8.34, -179.776694, 1.028973) (8.34, -174.253388, 0.627049) (8.34, -172.449614, -1.693332) (8.34, -171.00686, -3.768636) (8.34, -92.003508, -27.664773) on bodies 14 in component "Lowes Pipe Holder 6.75\""
sketch "Sketch2 (4)" plane through (0, -15.18853, -50.684001) normal (0, -0.287059, -0.957913) x (1, 0, 0) in component "Lowes Pipe Holder 6.75\""
  line L0 (7.32, 116.848716) -> (7.32, 101.848716)
  arc A0 (3.32, 101.848716) -> (7.32, 101.848716) centre (5.32, 101.848716) ccw
  line L1 (3.32, 101.848716) -> (3.32, 116.848716)
  arc A1 (7.32, 116.848716) -> (3.32, 116.848716) centre (5.32, 116.848716) ccw
  circle A2 centre (5.32, 41.848716) radius 2
  line L2 (-1.18, -3.651284) -> (11.82, -3.651284)
  line L3 (11.82, -3.651284) -> (11.82, 162.221023)
  line L4 (11.82, 162.221023) -> (-1.18, 162.221023)
  line L5 (-1.18, 162.221023) -> (-1.18, -3.651284)
  circle A3 centre (5.32, 41.848716) radius 1.7
  line L6 (5.32, 116.848716) -> (5.32, 101.848716) construction
  circle A4 centre (5.32, 109.348716) radius 1.7
  dimension "d210" = 3.4
  dimension "d211" = 3.4
  constraint concentric A2 A3
  measures "d210" diameter of A3
  measures "d211" diameter of A4
extrude "Extrude2''''''" cut sketch "Sketch2 (4)" against normal blind 10 contours A3 | A4 picked at (5.673311, 42.62581) picked at (4.344266, 109.818604) bodies 14 in component "Lowes Pipe Holder 6.75\""
sketch "Sketch1 (11)" plane through (0, 0, 0) normal (1, 0, 0) x (0, 1, 0) in component "Pipe"
  circle A0 centre (0, 0) radius 9.65
  circle A1 centre (0, 0) radius 8.65
  dimension "d147" = 19.3
  dimension "d148" = 17.3
  constraint coincident A0.centre A1.centre
  measures "d147" diameter of A0
  measures "d148" diameter of A1
extrude "Extrude1''''''''''" add sketch "Sketch1 (11)" along normal blind 2286 separate body contours A0 picked at (9.280739, -0.479419) makes body 15 in component "Pipe"
sketch "Sketch1 (12)" plane through (0, 0, 0) normal (1, 0, 0) x (0, 1, 0) in component "Shelf Board 10\" Depth"
  line L0 (0, 0) -> (-245.872, 0)
  line L1 (-245.872, 0) -> (-245.872, 16.002)
  line L2 (-245.872, 16.002) -> (0, 16.002)
  line L3 (0, 16.002) -> (0, 0)
  dimension "d156" = 245.872
  dimension "d157" = 16.002
  constraint horizontal L0
  constraint vertical L1
  constraint horizontal L2
  constraint vertical L3
  constraint coincident L0.start L3.end
  measures "d156" distance of L0.start L0.end
  measures "d157" distance of L0.start L2.end
extrude "Extrude1'''''''''''" add sketch "Sketch1 (12)" along normal blind 1828.8 separate body contours L0 L1 L2 L3 picked at (-163.914667, 5.334) makes body 16 in component "Shelf Board 10\" Depth"
pattern_linear "00000000-0000-0000-0000-000000000000" [suppressed]
sketch "Sketch1 (13)" plane through (0, 0, 0) normal (1, 0, 0) x (0, 1, 0) in component "Stone Harbor Pipe Holder 7\""
  line L0 (-172.821337, 14.828973) -> (-172.821337, 1.028973) construction
  line L1 (-16.821337, 12.828973) -> (-16.821337, -0.971027) construction
  circle A0 centre (-172.821337, 14.828973) radius 10.05
  circle A1 centre (-16.821337, 12.828973) radius 10.05
  line L2 (-30.621337, 0.028973) -> (-30.621337, 12.828973)
  circle A2 centre (-172.821337, 14.828973) radius 13.8
  line L3 (-3.021337, -51.040169) -> (-3.021337, 12.828973)
  circle A3 centre (-16.821337, 12.828973) radius 13.8
  line L4 (-159.021337, 14.828973) -> (-109.633858, 0.028973)
  line L5 (-172.821337, 14.828973) -> (-159.021337, 14.828973) construction
  line L6 (-160.169573, -3.947386) -> (-163.042675, 1.028973)
  line L7 (-163.042675, 1.028973) -> (-172.821337, 1.028973)
  line L8 (-30.621337, 0.028973) -> (-109.633858, 0.028973)
  line L9 (-3.021337, -51.040169) -> (-160.169573, -3.947386)
  line L10 (-8.021337, -11.171027) -> (-8.021337, -21.171027)
  line L11 (-8.021337, -21.171027) -> (-3.021337, -25.366525)
  line L12 (-3.021337, -6.975529) -> (-8.021337, -11.171027)
  point P0 (-8.021337, -16.171027)
  dimension "d168_1" = 20.1
  dimension "d169_1" = 27.6
  dimension "d170_1" = 20.1
  dimension "d171_1" = 27.6
  dimension "d216" = 63.869142
  dimension "d217" = 12.8
  dimension "d233" = 120
  dimension "d234" = 9.778663
  dimension "d235" = 5.746204
  dimension "d237" = 1
  dimension "d242" = 156
  dimension "d248" = 130
  dimension "d249" = 10
  dimension "d250" = 29
  constraint concentric A1 A3
  constraint concentric A0 A2
  constraint vertical L1
  constraint tangent L3 A3
  constraint vertical L3
  constraint vertical L2
  constraint tangent L2 A3
  constraint vertical L0
  constraint horizontal L5
  constraint tangent A2 L7
  constraint perpendicular L2 L8
  constraint horizontal L7
  constraint parallel L4 L9
  constraint equal L11 L12
  constraint vertical L10
  measures "d168_1" diameter of A1
  measures "d169_1" diameter of A3
  measures "d170_1" diameter of A0
  measures "d171_1" diameter of A2
  measures "d233" angle of L6 L7
  measures "d237" distance of L7 L8
  measures "d248" angle of L10 L12
extrude "Extrude1''''''''''''" add sketch "Sketch1 (13)" along normal blind 11 separate body contours L2 A2 L3 A3 L4 L6 L7 L8 L9 L10 L11 L12 | A3 | A2 picked at (-47.758844, -16.994075) picked at (-4.322715, 12.143378) picked at (-173.746643, 2.338128) makes body 17 in component "Stone Harbor Pipe Holder 7\""
move_face "OffsetFaces1''" offset -0.3 1 faces at (0, -47.758844, -16.994075) on bodies 17 in component "Stone Harbor Pipe Holder 7\""
move_face "OffsetFaces2''" offset -0.3 1 faces at (11, -47.758844, -16.994075) on bodies 17 in component "Stone Harbor Pipe Holder 7\""
fillet "Fillet1''''" radius 8 1 edges at (5.5, -30.621337, 0.028973) on bodies 17 in component "Stone Harbor Pipe Holder 7\""
fillet "Fillet2''''" radius 100 1 edges at (5.5, -109.633858, 0.028973) on bodies 17 in component "Stone Harbor Pipe Holder 7\""
fillet "Fillet3''''" radius 10 1 edges at (5.5, -159.021337, 14.828973) on bodies 17 in component "Stone Harbor Pipe Holder 7\""
fillet "Fillet4''''" radius 3 2 edges at (5.5, -163.042675, 1.028973) (5.5, -160.169573, -3.947386) on bodies 17 in component "Stone Harbor Pipe Holder 7\""
chamfer "Chamfer1''" distance 2 angle 45 30 edges at (0.3, -161.470951, -1.693332) (0.3, -160.028197, -3.768636) (0.3, -81.024845, -27.664773) (0.3, -3.021337, 2.926722) (0.3, -3.021337, -38.203347) (0.3, -16.821337, 26.628973) (0.3, -30.621337, 10.428973) (0.3, -32.964483, 2.372118) (0.3, -66.796862, 0.028973) (0.3, -109.478773, 1.086743) (0.3, -138.449421, 8.664164) (0.3, -157.261761, 15.442932) (0.3, -184.072551, 22.819603) (0.3, -168.798031, 1.028973) (0.3, -163.274725, 0.627049) (10.7, -161.470951, -1.693332) (10.7, -163.274725, 0.627049) (10.7, -168.798031, 1.028973) (10.7, -184.072551, 22.819603) (10.7, -157.261761, 15.442932) (10.7, -138.449421, 8.664164) (10.7, -109.478773, 1.086743) (10.7, -66.796862, 0.028973) (10.7, -32.964483, 2.372118) (10.7, -30.621337, 10.428973) (10.7, -16.821337, 26.628973) (10.7, -3.021337, -38.203347) (10.7, -3.021337, 2.926722) (10.7, -81.024845, -27.664773) (10.7, -160.028197, -3.768636) on bodies 17 in component "Stone Harbor Pipe Holder 7\""
fillet "Fillet5'''" radius 4 30 edges at (2.3, -161.470951, -1.693332) (2.3, -163.274725, 0.627049) (2.3, -168.798031, 1.028973) (2.3, -184.072551, 22.819603) (2.3, -157.261761, 15.442932) (2.3, -138.449421, 8.664164) (2.3, -109.478773, 1.086743) (2.3, -66.796862, 0.028973) (2.3, -32.964483, 2.372118) (2.3, -30.621337, 10.428973) (2.3, -16.821337, 26.628973) (2.3, -3.021337, 2.926722) (2.3, -3.021337, -38.203347) (2.3, -160.028197, -3.768636) (2.3, -81.024845, -27.664773) (8.7, -3.021337, -38.203347) (8.7, -3.021337, 2.926722) (8.7, -16.821337, 26.628973) (8.7, -30.621337, 10.428973) (8.7, -32.964483, 2.372118) (8.7, -66.796862, 0.028973) (8.7, -109.478773, 1.086743) (8.7, -138.449421, 8.664164) (8.7, -157.261761, 15.442932) (8.7, -184.072551, 22.819603) (8.7, -168.798031, 1.028973) (8.7, -163.274725, 0.627049) (8.7, -161.470951, -1.693332) (8.7, -160.028197, -3.768636) (8.7, -81.024845, -27.664773) on bodies 17 in component "Stone Harbor Pipe Holder 7\""